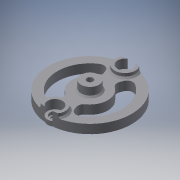
# Autodesk Inventor part: small_magnet_holder5
Saved by Autodesk Inventor 2017 SP1 (Build 210196100, 196)
## iProperties
Part Number: small_magnet_holder5
Material: Générique
Document SubType Name: Modeling
Designer: tmonglon
Density: 1 g/cm^3
Appearance: Par défaut
Author: tmonglon
Autodesk Inventor part; units mm, degrees
ref_plane "YZ Plane" through (0, 0, 0) normal (1, 0, 0) x (0, 1, 0)
ref_plane "XZ Plane" through (0, 0, 0) normal (0, 1, 0) x (-1, 0, 0)
ref_plane "XY Plane" through (0, 0, 0) normal (0, 0, 1) x (1, 0, 0)
sketch "Esquisse1" plane through (0, 0, 0) normal (0, 0, 1) x (1, 0, 0)
  circle A0 centre (0, 0) radius 1.05
  circle A1 centre (0, 0) radius 3
  circle A2 centre (0, 11.8) radius 1.7
  circle A3 centre (0, 11.8) radius 2.5
  circle A4 centre (0, -11.8) radius 2.5
  circle A5 centre (0, -11.8) radius 1.7
  circle A6 centre (0, 11.8) radius 1.25
  circle A7 centre (0, -11.8) radius 1.25
  arc A8 (-1.292, 13.9403) -> (-1.292, -13.9403) centre (0, 0) ccw
  arc A9 (1.292, -13.9403) -> (1.292, 13.9403) centre (0, 0) ccw
  dimension "d1" = 2.1
  dimension "d2" = 6
  dimension "d3" = 3.4
  dimension "d4" = 11.8
  dimension "d5" = 5
  dimension "d8" = 360
  dimension "d12" = 2.5
  dimension "d15" = 360
  constraints: 10 centre point, 8 point on circle, 6 coincident, 14 other
  measures "d1" diameter of A0
  measures "d2" diameter of A1
  measures "d3" diameter of A2
  measures "d4" distance of A2.centre point (0, 0)
  measures "d5" diameter of A3
  measures "d12" diameter of A6
extrude "Extrusion10" add sketch "Esquisse1" along normal blind 3 contours A3 A9 A4 A8
extrude "Extrusion11" add sketch "Esquisse1" along normal blind 6 contours A1
extrude "Extrusion12" add sketch "Esquisse1" along normal blind 0.5 contours A2 | A5
extrude "Extrusion13" add sketch "Esquisse1" along normal blind 1.5 contours A3 | A4
sketch "Esquisse3" plane through (0, 0, 3) normal (0, 0, 1) x (1, 0, 0)
  circle A0 centre (0, 0) radius 1.05 projected
  line L0 (0, 0) -> (-7.6468, 0)
  circle A1 centre (0, 0) radius 3 projected
  line L1 (0, 0) -> (4.4865, 0)
  line L2 (0, 16.0443) -> (0, -15.4592)
  line L3 (0, 0) -> (-3.7622, -10.3366)
  line L4 (0, 0) -> (3.7622, -10.3366)
  line L5 (0, 0) -> (3.7622, 10.3366)
  line L6 (0, 0) -> (-3.7622, 10.3366)
  arc A2 (3.7622, -10.3366) -> (3.7622, 10.3366) centre (0, 0) ccw
  arc A3 (-3.7622, 10.3366) -> (-3.7622, -10.3366) centre (0, 0) ccw
  arc A4 (2.0521, -5.6382) -> (2.0521, 5.6382) centre (0, 0) ccw
  arc A5 (-2.0521, 5.6382) -> (-2.0521, -5.6382) centre (0, 0) ccw
  dimension "d75" = 360
  dimension "d71" = 20
  dimension "d72" = 40
  constraints: 14 end point, 8 point on circle, 5 point on line, 4 centre point, 2 coincident, 1 horizontal, 1 vertical, 11 other
  measures "d71" angle of L3 L2
  measures "d72" angle of L4 L3
extrude "Extrusion15" cut sketch "Esquisse3" against normal through all contours L5 A2 L4 A4 | A5 L3 A3 L6
fillet "Congé1" radius 2 8 edges at (3.7622, -10.3366, 1.5) (-3.7622, -10.3366, 1.5) (-3.7622, 10.3366, 1.5) (3.7622, 10.3366, 1.5) (-2.0521, -5.6382, 1.5) (-2.0521, 5.6382, 1.5) (2.0521, -5.6382, 1.5) (2.0521, 5.6382, 1.5)
chamfer "Chanfrein1" distance 0.5 angle 45 1 edges at (-3, 0, 3)
sketch "Esquisse4" plane through (0, 0, 3) normal (0, 0, 1) x (1, 0, 0)
  arc A0 (-1.292, 13.9403) -> (1.292, 13.9403) centre (0, 11.8) ccw projected
  arc A1 (-1.292, 13.9403) -> (-1.292, -13.9403) centre (0, 0) ccw projected
  arc A2 (1.292, -13.9403) -> (-1.292, -13.9403) centre (0, -11.8) ccw projected
  arc A3 (1.292, -13.9403) -> (1.292, 13.9403) centre (0, 0) ccw projected
  line L0 (-2.6493, -7.2788) -> (-3.0012, -8.2458) projected
  arc A4 (-5.9652, -9.2421) -> (-3.0012, -8.2458) centre (-4.8806, -7.5617) ccw projected
  arc A5 (-5.9652, 9.2421) -> (-5.9652, -9.2421) centre (0, 0) ccw projected
  arc A6 (-3.0012, 8.2458) -> (-5.9652, 9.2421) centre (-4.8806, 7.5617) ccw projected
  line L1 (-3.0012, 8.2458) -> (-2.6493, 7.2788) projected
  arc A7 (-3.3965, 4.9461) -> (-2.6493, 7.2788) centre (-4.5287, 6.5948) ccw projected
  arc A8 (-3.3965, 4.9461) -> (-3.3965, -4.9461) centre (0, 0) ccw projected
  arc A9 (-2.6493, -7.2788) -> (-3.3965, -4.9461) centre (-4.5287, -6.5948) ccw projected
  line L2 (2.6493, 7.2788) -> (3.0012, 8.2458) projected
  arc A10 (5.9652, 9.2421) -> (3.0012, 8.2458) centre (4.8806, 7.5617) ccw projected
  arc A11 (5.9652, -9.2421) -> (5.9652, 9.2421) centre (0, 0) ccw projected
  arc A12 (3.0012, -8.2458) -> (5.9652, -9.2421) centre (4.8806, -7.5617) ccw projected
  line L3 (3.0012, -8.2458) -> (2.6493, -7.2788) projected
  arc A13 (3.3965, -4.9461) -> (2.6493, -7.2788) centre (4.5287, -6.5948) ccw projected
  arc A14 (3.3965, -4.9461) -> (3.3965, 4.9461) centre (0, 0) ccw projected
  arc A15 (2.6493, 7.2788) -> (3.3965, 4.9461) centre (4.5287, 6.5948) ccw projected
  circle A16 centre (0, 0) radius 3.5 projected
  arc A17 (2.9484, -13.686) -> (-2.9484, -13.686) centre (0, -11.8) ccw
  circle A18 centre (0, 11.8) radius 3.5
  arc A19 (-1.292, 13.9403) -> (-1.292, -13.9403) centre (0, 0) ccw projected
  arc A20 (1.292, -13.9403) -> (-1.292, -13.9403) centre (0, -11.8) ccw projected
  arc A21 (1.292, -13.9403) -> (1.292, 13.9403) centre (0, 0) ccw projected
  line L4 (2.9484, -13.686) -> (1.292, -13.9403)
  dimension "d84" = 7
  dimension "d85" = 7
  dimension "d94" = 2.5
  constraints: 5 point on circle, 2 centre point, 2 coincident, 2 end point
  measures "d84" diameter of A17
  measures "d85" diameter of A18
  measures "d94" radius of A0
extrude "Extrusion16" add sketch "Esquisse4" along normal blind 1.5 contours A17 L4 A2 A1
chamfer "Chanfrein2" distance 0.5 angle 45 1 edges at (0, -8.3, 3)
pattern_circular "Réseau circulaire2" count 2 over 360 about axis through (0, 0, 0) along (0, 0, 1) of "Extrusion16", "Chanfrein2"
